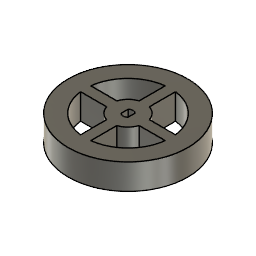
ensamble avance 2 (1) (Autodesk Fusion 360 archive; units mm, degrees)
design "rueda"
Autodesk Fusion 360 part; units mm, degrees
sketch "Boceto1" plane through (0, 0, 0) normal (0, 0, 1) x (1, 0, 0)
  circle A0 centre (0, 0) radius 35
  line L0 (3, 24.8193) -> (3, 9.5394)
  line L1 (-3, 24.8193) -> (-3, 9.5394)
  line L2 (3, -24.8193) -> (3, -9.5394)
  line L3 (-3, -24.8193) -> (-3, -9.5394)
  line L4 (-24.8193, 3) -> (-9.5394, 3)
  line L5 (-24.8193, -3) -> (-9.5394, -3)
  line L6 (9.5385, -3.0027) -> (24.819, -3.0027)
  line L7 (9.5394, 3) -> (24.8193, 3)
  arc A1 (-3, 9.5394) -> (-9.5394, 3) centre (0, 0) ccw
  arc A2 (9.5394, 3) -> (3, 9.5394) centre (0, 0) ccw
  arc A3 (-9.5394, -3) -> (-3, -9.5394) centre (0, 0) ccw
  arc A4 (3, -9.5394) -> (9.5385, -3.0027) centre (0, 0) ccw
  arc A5 (-24.8193, -3) -> (-3, -24.8193) centre (0, 0) ccw
  arc A6 (3, -24.8193) -> (24.819, -3.0027) centre (0, 0) ccw
  arc A7 (24.8193, 3) -> (3, 24.8193) centre (0, 0) ccw
  arc A8 (-3, 24.8193) -> (-24.8193, 3) centre (0, 0) ccw
  line L8 (2, 0) -> (2, 2.1)
  line L9 (-2, 2.1) -> (-2, -2.1)
  line L10 (2, -2.1) -> (2, 0)
  arc A9 (-2, -2.1) -> (2, -2.1) centre (0, 0) ccw
  arc A10 (2, 2.1) -> (-2, 2.1) centre (0, 0) ccw
  dimension "d1" = 50
  dimension "d2" = 20
  dimension "d3" = 2
  dimension "d4" = 2.1
  dimension "d5" = 4
  dimension "d6" = 4.2
  constraint coincident A0.centre A1.centre
  constraint concentric A0 A5
  constraint parallel L5 L6
  constraint parallel L4 L7
  constraint concentric A1 A3
  constraint concentric A2 A4
  constraint concentric A3 A4
  constraint concentric A5 A6
  constraint concentric A6 A7
  constraint concentric A7 A8
  constraint concentric A4 A9
  constraint concentric A9 A10
  measures "d1" diameter of A5
  measures "d2" diameter of A3
  measures "d3" distance of A0.centre L8.start
  measures "d4" distance of L8.start L8.end
  measures "d5" distance of L8.end L9.start
  measures "d6" distance of L9.start L9.end
extrude "Extruir1" add sketch "Boceto1" along normal blind 15

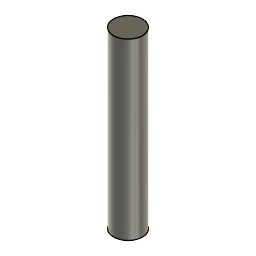
design "pasador 5mm"
Autodesk Fusion 360 part; units mm, degrees
sketch "Boceto1" plane through (0, 0, 0) normal (0, 0, 1) x (1, 0, 0)
  circle A0 centre (0, 0) radius 2.5
  dimension "d1" = 5
  constraint coincident A0.centre origin
  measures "d1" diameter of A0
extrude "Extruir1" add sketch "Boceto1" along normal blind 30
